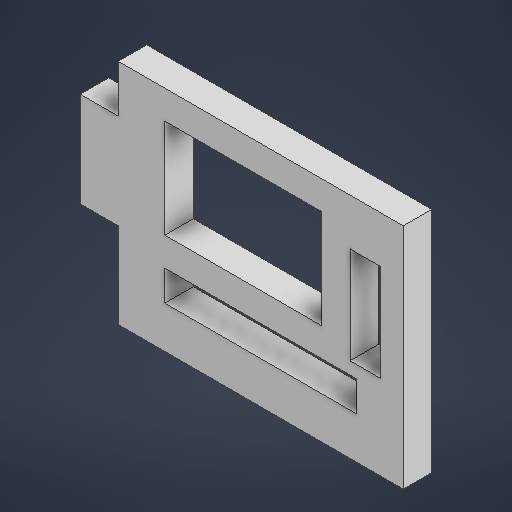
# Autodesk Inventor part: Battary_holder
Saved by Autodesk Inventor 2027 (Build 310192000, 192)
## iProperties
Created: 2026-05-15
Part Number: Battary_holder
Material: Generic
Document SubType Name: Modeling
Designer: alexy
Density: 1 g/cm^3
Appearance: Default
Author: alexy
Autodesk Inventor part; units mm, degrees
ref_plane "YZ Plane" through (0, 0, 0) normal (1, 0, 0) x (0, 1, 0)
ref_plane "XZ Plane" through (0, 0, 0) normal (0, 1, 0) x (-1, 0, 0)
ref_plane "XY Plane" through (0, 0, 0) normal (0, 0, 1) x (1, 0, 0)
sketch "Sketch1" plane through (0, 0, 0) normal (0, 0, 1) x (1, 0, 0)
  line L0 (0, 9) -> (-4, 9)
  line L1 (-4, 9) -> (-4, 19)
  line L2 (-4, 19) -> (0, 19)
  line L3 (0, 19) -> (0, 9)
  line L4 (0, 9) -> (0, 0)
  line L5 (0, 0) -> (30, 0)
  line L6 (30, 0) -> (30, 24)
  line L7 (30, 24) -> (0, 24)
  line L8 (0, 24) -> (0, 19)
  line L9 (4.9, 7.6) -> (25.1, 7.6)
  line L10 (25.1, 7.6) -> (25.1, 4.4)
  line L11 (25.1, 4.4) -> (4.9, 4.4)
  line L12 (4.9, 4.4) -> (4.9, 7.6)
  line L13 (4.9, 7.6) -> (25.1, 4.4) construction
  line L14 (25.1, 7.6) -> (4.9, 4.4) construction
  line L15 (24.4, 19.1) -> (27.6, 19.1)
  line L16 (27.6, 19.1) -> (27.6, 8.9)
  line L17 (27.6, 8.9) -> (24.4, 8.9)
  line L18 (24.4, 8.9) -> (24.4, 19.1)
  line L19 (24.4, 19.1) -> (27.6, 8.9) construction
  line L20 (27.6, 19.1) -> (24.4, 8.9) construction
  line L21 (34, 19) -> (30, 19)
  line L22 (30, 19) -> (30, 9)
  line L23 (30, 9) -> (34, 9)
  line L24 (34, 9) -> (34, 19)
  line L25 (34, 19) -> (30, 9) construction
  line L26 (30, 19) -> (34, 9) construction
  point P0 (15, 6)
  point P1 (15, 0)
  point P2 (26, 14)
  point P3 (0, 14)
  point P4 (32, 14)
  dimension "d0" = 10
  dimension "d1" = 4
  dimension "d4" = 30
  dimension "d5" = 20.2
  dimension "d6" = 3.2
  dimension "d8" = 6
  dimension "d11" = 3.2
  dimension "d12" = 4
  dimension "d13" = 10.2
  dimension "d20" = 4
  dimension "d21" = 24
  dimension "d22" = 9
  constraints: 54 end point, 8 midpoint, 8 parallel, 8 perpendicular, 4 horizontal, 3 horizontal alignment, 2 point on line, 2 vertical alignment, 1 vertical
  measures "d0" distance of L0.end L1.end
  measures "d1" distance of L1.end L2.end
  measures "d4" distance of L4.end L5.end
  measures "d5" distance of L10.end L11.end
  measures "d6" distance of L9.end L10.end
  measures "d8" vertical distance of L4.end point (15, 6)
  measures "d11" distance of L15.start L15.end
  measures "d12" distance from line of L6 point (26, 14)
  measures "d13" distance of L15.end L16.end
  measures "d20" distance of L21.start L21.end
  measures "d21" distance of L5.end L6.end
  measures "d22" distance from line of L4.end L0
extrude "Extrusion1" add sketch "Sketch1" along normal blind 3 contours L0 L1 L2 L3 | L3 L8 L7 L6 L5 L4
sketch "Sketch2" plane through (0, 0, 3) normal (0, 0, 1) x (1, 0, 0)
  line L0 (4.9, 21) -> (21.4, 21)
  line L1 (21.4, 21) -> (21.4, 10.6)
  line L2 (21.4, 10.6) -> (4.9, 10.6)
  line L3 (4.9, 10.6) -> (4.9, 21)
  line L4 (24.4, 8.9) -> (24.4, 19.1) projected
  line L5 (4.9, 7.6) -> (25.1, 7.6) projected
  line L6 (30, 24) -> (0, 24) projected
  line L7 (0, 9) -> (0, 0) projected
  dimension "d14" = 3
  dimension "d15" = 3
  dimension "d16" = 3
  constraints: 8 end point, 2 parallel, 1 horizontal, 1 perpendicular, 1 vertical alignment
  measures "d14" distance between parallel lines of L4 L1
  measures "d15" distance between parallel lines of L5 L2
  measures "d16" distance between parallel lines of L6 L0
extrude "Extrusion2" cut sketch "Sketch2" against normal blind 3
body "Solid1"
